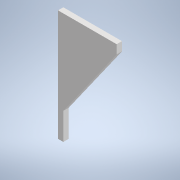
# Autodesk Inventor part: Side
Saved by Autodesk Inventor 2021 (Build 250183000, 183)
## iProperties
Created: 2020-07-16
Part Number: Side
Material: Generic
Document SubType Name: Modeling
Designer: adick
Density: 1 g/cm^3
Appearance: Default
Author: adick
Autodesk Inventor part; units mm, degrees
ref_plane "YZ Plane" through (0, 0, 0) normal (1, 0, 0) x (0, 1, 0)
ref_plane "XZ Plane" through (0, 0, 0) normal (0, 1, 0) x (-1, 0, 0)
ref_plane "XY Plane" through (0, 0, 0) normal (0, 0, 1) x (1, 0, 0)
sketch "Sketch1" plane through (0, 0, 0) normal (0, 0, 1) x (1, 0, 0)
  line L0 (6.35, -132.5) -> (19.05, -132.5)
  line L1 (19.05, 132.5) -> (6.35, 132.5)
  line L2 (6.35, 132.5) -> (6.35, -132.5)
  line L3 (146.05, 111.3788) -> (146.05, 132.5)
  line L4 (146.05, 132.5) -> (19.05, 132.5)
  line L5 (146.05, 111.3788) -> (19.05, -68.2625)
  line L6 (19.05, -132.5) -> (19.05, -68.2625)
  point P0 (0, 0)
  constraints: 14 end point, 2 parallel, 1 horizontal, 1 perpendicular, 2 other
extrude "Extrusion1" add sketch "Sketch1" against normal blind 12.7
body "Solid1"
